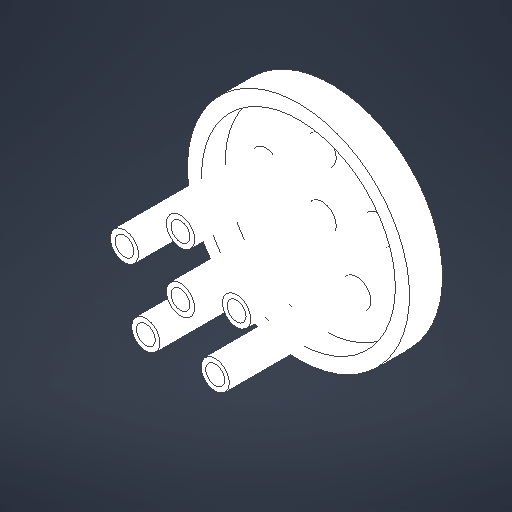
# Autodesk Inventor part: TAPA CAPSULA
Saved by Autodesk Inventor 2026.2 (Build 302298000, 298)
## iProperties
Created: 2025-12-31
Part Number: TAPA CAPSULA
Material: Genérico
Document SubType Name: Modeling
Designer: vicho
Density: 1 g/cm^3
Appearance: Valor por defecto
Author: vicho
Autodesk Inventor part; units mm, degrees
ref_plane "YZ Plane" through (0, 0, 0) normal (1, 0, 0) x (0, 1, 0)
ref_plane "XZ Plane" through (0, 0, 0) normal (0, 1, 0) x (-1, 0, 0)
ref_plane "XY Plane" through (0, 0, 0) normal (0, 0, 1) x (1, 0, 0)
sketch "Boceto1" plane through (0, 0, 0) normal (0, 0, 1) x (1, 0, 0)
  line L0 (0, 55.4788) -> (0, -87.4245) construction
  line L1 (-101.2305, 0) -> (87.3085, 0) construction
  circle A0 centre (0, 0) radius 23.525
  dimension "d0" = 47.05
  constraints: 4 end point, 2 point on line, 1 centre point, 1 coincident, 1 horizontal, 1 vertical
  measures "d0" diameter of A0
extrude "Extrusión1" add sketch "Boceto1" along normal blind 7
sketch "Boceto2" plane through (0, 0, 7) normal (0, 0, 1) x (1, 0, 0)
  circle A0 centre (0, 0) radius 20.525
  dimension "d3" = 41.05
  constraints: 1 centre point, 1 coincident
  measures "d3" diameter of A0
extrude "Extrusión2" cut sketch "Boceto2" against normal blind 5
sketch "Boceto4" plane through (0, 0, 2) normal (0, 0, 1) x (1, 0, 0)
  line L0 (0, 23.5497) -> (0, -28.0756) construction
  line L1 (-25.4254, 0) -> (29.9443, 0) construction
  circle A0 centre (0, 0) radius 3
  circle A1 centre (0, 0) radius 12.5 construction
  circle A2 centre (0, 12.5) radius 3
  circle A3 centre (-11.8882, 3.8627) radius 3
  circle A4 centre (-7.3473, -10.1127) radius 3
  circle A5 centre (7.3473, -10.1127) radius 3
  circle A6 centre (11.8882, 3.8627) radius 3
  dimension "d16" = 25
  dimension "d15" = 6
  dimension "d17" = 6
  dimension "d20" = 360
  constraints: 6 centre point, 4 end point, 3 point on line, 2 coincident, 1 horizontal, 1 vertical, 1 vertical alignment, 13 other
  measures "d15" diameter of A0
  measures "d17" diameter of A2
extrude "Extrusión4" add sketch "Boceto4" along normal blind 30
sketch "Boceto5" plane through (0, 0, 32) normal (0, 0, 1) x (1, 0, 0)
  circle A0 centre (0, 0) radius 2
  circle A1 centre (-11.8882, 3.8627) radius 3 projected
  circle A2 centre (-11.8882, 3.8627) radius 2
  circle A3 centre (-7.3473, -10.1127) radius 2
  circle A4 centre (7.3473, -10.1127) radius 2
  circle A5 centre (11.8882, 3.8627) radius 2
  circle A6 centre (0, 12.5) radius 2
  dimension "d24" = 4
  dimension "d25" = 4
  dimension "d28" = 360
  constraints: 6 centre point, 2 coincident, 11 other
  measures "d24" diameter of A0
  measures "d25" diameter of A2
extrude "Extrusión5" cut sketch "Boceto5" against normal blind 40 contours A0 | A2 | A3 | A4 | A5 | A6
